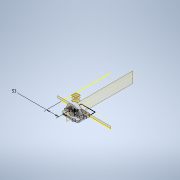
# Autodesk Inventor part: CameraHolder
Saved by Autodesk Inventor 2022 (Build 260153000, 153)
## iProperties
Created: 2024-03-25
Part Number: CameraHolder
Material: Generic
Document SubType Name: Modeling
Designer: Gotham City
Density: 1 g/cm^3
Appearance: Default
Author: Gotham City
Autodesk Inventor part; units mm, degrees
ref_plane "XY Plane" through (0, 0, 0) normal (0, 0, 1) x (1, 0, 0)
ref_plane "GlassTop" through (0, 0, 0) normal (0, 1, 0) x (-1, 0, 0)
ref_plane "CameraFocus" through (0, 1.5, 0) normal (0, 1, 0) x (-1, 0, 0)
ref_plane "HeatbedMountTop" through (0, -18, 0) normal (0, 1, 0) x (-1, 0, 0)
ref_plane "HeatbedBottom" through (0, -8, 0) normal (0, 1, 0) x (-1, 0, 0)
ref_plane "CameraBottom" through (0, -18.5, 0) normal (0, 1, 0) x (-1, 0, 0)
sketch "Sketch1" plane through (0, -18, 0) normal (0, 1, 0) x (-1, 0, 0)
  line L0 (-144, 0) -> (0, 0)
  line L1 (0, 0) -> (0, -144)
  line L2 (0, -144) -> (-144, -144)
  line L3 (-144, -144) -> (-144, 0)
  circle A0 centre (-11, -11) radius 2.5
  line L4 (-39.5, -4) -> (-24, -4)
  line L5 (-24, -4) -> (-24, -11.5)
  line L6 (-24, -11.5) -> (-39.5, -11.5)
  line L7 (-39.5, -11.5) -> (-39.5, -4)
  line L8 (-59.5, -4) -> (-44, -4)
  line L9 (-44, -4) -> (-44, -11.5)
  line L10 (-44, -11.5) -> (-59.5, -11.5)
  line L11 (-59.5, -11.5) -> (-59.5, -4)
  line L12 (-79.5, -4) -> (-64, -4)
  line L13 (-64, -4) -> (-64, -11.5)
  line L14 (-64, -11.5) -> (-79.5, -11.5)
  line L15 (-79.5, -11.5) -> (-79.5, -4)
  line L16 (-15.5, -44) -> (-8, -44)
  line L17 (-8, -44) -> (-8, -59.5)
  line L18 (-8, -59.5) -> (-15.5, -59.5)
  line L19 (-15.5, -59.5) -> (-15.5, -44)
  line L20 (-15.5, -79.5) -> (-15.5, -64)
  line L21 (-8, -64) -> (-8, -79.5)
  line L22 (-8, -79.5) -> (-15.5, -79.5)
  line L23 (-15.5, -64) -> (-8, -64)
  line L24 (-15.5, -99.5) -> (-15.5, -84)
  line L25 (-8, -84) -> (-8, -99.5)
  line L26 (-8, -99.5) -> (-15.5, -99.5)
  line L27 (-15.5, -84) -> (-8, -84)
  circle A1 centre (-11, -35) radius 2.5
  point P0 (0, 0)
  dimension "d5" = 144
  dimension "d6" = 144
  dimension "d7" = 11
  dimension "d8" = 11
  dimension "d9" = 5
  dimension "d10" = 7.5
  dimension "d11" = 15.5
  dimension "d12" = 4
  dimension "d13" = 24
  dimension "d16" = 20
  dimension "d21" = 7.5
  dimension "d22" = 15.5
  dimension "d23" = 8
  dimension "d24" = 44
  dimension "d27" = 20
  dimension "d32" = 5
  dimension "d33" = 24
  constraints: 56 end point, 6 parallel, 4 horizontal, 3 perpendicular, 2 centre point, 2 collinear, 1 coincident, 1 vertical, 1 vertical alignment, 30 other
  measures "d5" distance of L0.start L0.end
  measures "d6" distance of L0.end L1.end
  measures "d7" distance from line of L0 A0.centre
  measures "d8" distance from line of L1 A0.centre
  measures "d9" diameter of A0
  measures "d10" distance of L6.end L4.start
  measures "d11" distance of L4.start L4.end
  measures "d12" distance between parallel lines of L0 L4
  measures "d13" distance between parallel lines of L1 L5
  measures "d16" distance of L4.start L8.start
  measures "d21" distance of L16.start L16.end
  measures "d22" distance of L16.end L17.end
  measures "d23" distance between parallel lines of L1 L17
  measures "d24" distance between parallel lines of L0 L16
  measures "d27" distance of L16.start L20.end
  measures "d32" diameter of A1
  measures "d33" distance of A0.centre A1.centre
extrude "Extrusion1" add sketch "Sketch1" against normal blind 2
sketch "Sketch2" plane through (0, 0, 0) normal (0, 1, 0) x (-1, 0, 0)
  line L0 (30.5, -184.5) -> (-184.5, -184.5)
  line L1 (-184.5, -184.5) -> (-184.5, 30.5)
  line L2 (-184.5, 30.5) -> (30.5, 30.5)
  line L3 (30.5, 30.5) -> (30.5, -184.5)
  circle A0 centre (-11, -11) radius 2.5 construction
  point P0 (0, 0)
  dimension "d36" = 215
  dimension "d37" = 215
  dimension "d38" = 41.5
  dimension "d39" = 41.5
  constraints: 8 end point, 2 parallel, 1 horizontal, 1 perpendicular
  measures "d36" distance of L0.end L1.end
  measures "d37" distance of L0.start L0.end
  measures "d38" distance from line of L2 A0.centre
  measures "d39" distance from line of L3 A0.centre
extrude "Extrusion2" add sketch "Sketch2" against normal up to surface (8 mm away) separate body
ref_plane "MaxCameraFront" through (-30.5, 0, 40.5) normal (0, 0, 1) x (1, 0, 0)
sketch "Sketch4" plane through (0, -20, 0) normal (0, 1, 0) x (-1, 0, 0)
  line L0 (-84.5, 0) -> (-22.5, 0) construction
  line L1 (-22.5, 0) -> (-22.5, 53.5)
  line L2 (-22.5, 53.5) -> (-84.5, 53.5)
  line L3 (-84.5, 53.5) -> (-84.5, 0)
  line L4 (-84.5, 0) -> (-84.5, 0) construction
  line L5 (-22.5, 0) -> (-84.5, 0)
  line L6 (-184.5, 30.5) -> (30.5, 30.5) projected
  line L7 (30.5, 30.5) -> (30.5, -184.5) projected
  circle A0 centre (-38, 44.5) radius 1.5
  circle A1 centre (-38, 33) radius 1.5
  circle A2 centre (-76, 44.5) radius 1.5
  circle A3 centre (-76, 33) radius 1.5
  line L8 (-53.5, 53.5) -> (-53.5, 0) construction
  line L9 (-144, 0) -> (0, 0) construction
  dimension "d58" = 23
  dimension "d59" = 53
  dimension "d60" = 62
  dimension "d61" = 14
  dimension "d62" = 11.5
  dimension "d63" = 3
  dimension "d64" = 3
  dimension "d65" = 15.5
  dimension "d66" = 3
  dimension "d67" = 38
  dimension "d68" = 3
  constraints: 14 end point, 4 centre point, 3 perpendicular, 2 horizontal, 2 horizontal alignment, 2 point on line, 2 vertical alignment, 1 midpoint, 1 parallel, 1 vertical
  measures "d58" distance between parallel lines of L6 L2
  measures "d59" distance between parallel lines of L7 L1
  measures "d60" distance between parallel lines of L3 L1
  measures "d61" distance from line of L6 A0.centre
  measures "d62" distance of A0.centre A1.centre
  measures "d63" diameter of A0
  measures "d64" diameter of A1
  measures "d65" distance from line of L1 A0.centre
  measures "d66" diameter of A2
  measures "d67" distance of A0.centre A2.centre
  measures "d68" diameter of A3
extrude "Extrusion3" add sketch "Sketch4" against normal blind 3 separate body
ref_plane "CameraSideCenter" through (53.5, -20, 53.5) normal (1, 0, 0) x (0, 1, 0)
sketch "Sketch3" plane through (53.5, 0, -184.5) normal (-1, 0, 0) x (0, 0, 1)
  line L0 (-53, 1.5) -> (318, 1.5) construction
  line L1 (225, 29.8) -> (225, -28.3) construction
  circle A0 centre (245, 1.5) radius 20 construction
  line L2 (245, 21.5) -> (245, -18.5)
  arc A1 (245, 21.5) -> (245, -18.5) centre (245, 1.5) ccw
  point P0 (184.5, 0)
  dimension "d47" = 40
  constraints: 4 point on circle, 2 centre point, 2 end point, 2 tangent, 1 midpoint, 1 point on line, 1 vertical
  measures "d47" diameter of A0
revolve "Revolution1" add sketch "Sketch3" angle 360 about axis through (53.5, 21.5, 60.5) along (0, -1, 0) separate body
sketch "Sketch6" plane through (0, -20, 0) normal (0, 1, 0) x (1, 0, 0)
  line L0 (17.5, -81.5) -> (89.5, -81.5)
  line L1 (89.5, -81.5) -> (89.5, -25.5)
  line L2 (89.5, -25.5) -> (17.5, -25.5)
  line L3 (17.5, -25.5) -> (17.5, -81.5)
  circle A0 centre (53.5, -60.5) radius 20 construction
  circle A1 centre (38, -33) radius 1.5 construction
  line L4 (33.5, -81.5) -> (33.5, -25.5) construction
  line L5 (73.5, -81.5) -> (73.5, -25.5) construction
  line L6 (17.5, -31.5) -> (89.5, -31.5) construction
  line L7 (17.5, -80.5) -> (95.4239, -80.5) construction
  point P0 (0, 0)
  dimension "d69" = 16
  dimension "d70" = 16
  dimension "d71" = 1
  dimension "d72" = 6
  constraints: 16 end point, 7 point on line, 5 perpendicular, 4 tangent, 2 parallel, 1 horizontal
  measures "d69" distance between parallel lines of L3 L4
  measures "d70" distance between parallel lines of L1 L5
  measures "d71" distance between parallel lines of L7 L0
  measures "d72" distance between parallel lines of L6 L2
extrude "Extrusion5" add sketch "Sketch6" along normal blind 8 separate body
revolve "Revolution3" cut sketch "Sketch3" angle 360 about axis through (53.5, 21.5, 60.5) along (0, -1, 0) bodies 5
sketch "Sketch7" plane through (0, -12, 0) normal (0, 1, 0) x (1, 0, 0)
  circle A0 centre (76, -44.5) radius 1.5 projected
  circle A1 centre (76, -33) radius 1.5 projected
  circle A2 centre (38, -44.5) radius 1.5 projected
  circle A3 centre (38, -33) radius 1.5 projected
  point P0 (0, 0)
hole "Hole1" at (76, -12, 33) at (76, -12, 44.5) at (38, -12, 44.5) at (38, -12, 33) direction (0, -1, 0) diameter 2.6 end through all counterbore diameter 5.5 counterbore depth 2 bodies 5 clearance for "Socket Head Cap Screw ISO 4762" size "M2.5" standard "ISO"
sketch "Sketch8" plane through (0, -12, 0) normal (0, 1, 0) x (1, 0, 0)
  line L0 (17.5, -25.5) -> (17.5, -81.5) construction
  line L1 (89.5, -81.5) -> (89.5, -25.5) construction
  line L2 (89.5, -81.5) -> (89.5, -25.5) projected
  line L3 (17.5, -52.5) -> (89.5, -52.5)
  line L4 (89.5, -52.5) -> (89.5, -68.5)
  line L5 (89.5, -68.5) -> (17.5, -68.5)
  line L6 (17.5, -68.5) -> (17.5, -52.5)
  circle A0 centre (53.5, -60.5) radius 20 construction
  line L7 (53.5, -60.5) -> (89.5, -60.5) construction
  point P0 (0, 0)
  dimension "d83" = 16
  constraints: 10 end point, 2 horizontal, 2 parallel, 2 point on line, 1 midpoint, 1 perpendicular
  measures "d83" distance between parallel lines of L5 L3
extrude "Extrusion6" add sketch "Sketch8" along normal blind 40 separate body
revolve "Revolution4" cut sketch "Sketch3" angle 360 about axis through (53.5, 21.5, 60.5) along (0, -1, 0) bodies 6
sketch "Sketch9" plane through (17.5, 28, 68.5) normal (0, 0, 1) x (1, 0, 0)
  arc A0 (48.3996, -40) -> (23.6004, -40) centre (36, -26.5) ccw construction
  line L0 (55.75, -40) -> (61.25, -40) projected
  line L1 (36, -26.5) -> (54.3303, -26.5)
  line L2 (54.3303, -26.5) -> (54.3303, -40)
  line L3 (54.3303, -40) -> (36, -40)
  line L4 (36, -40) -> (36, -26.5) construction
  line L5 (36, -26.5) -> (17.6697, -26.5)
  line L6 (17.6697, -26.5) -> (17.6697, -40)
  line L7 (17.6697, -40) -> (36, -40)
  point P0 (-17.5, -28)
  point P1 (55.75, -40)
  constraints: 14 end point, 2 parallel, 2 symmetric about line, 1 horizontal, 1 perpendicular, 1 point on circle, 1 point on line
extrude "Extrusion7" cut sketch "Sketch9" against normal through all bodies 6
sketch "Sketch10" plane through (17.5, 28, 68.5) normal (0, 0, 1) x (1, 0, 0)
  arc A0 (48.3996, -40) -> (23.6004, -40) centre (36, -26.5) ccw construction
  arc A1 (62.3303, -26.5) -> (9.6697, -26.5) centre (36, -26.5) ccw
  line L0 (0, -40) -> (0, 0) projected
  line L1 (0, -32) -> (0, 0)
  line L2 (0, 0) -> (72, 0) projected
  line L3 (36, 1.8) -> (36, -56.3) construction
  line L4 (72, -32) -> (72, 0)
  line L5 (9.6697, -26.5) -> (9.6697, -32)
  line L6 (9.6697, -32) -> (0, -32)
  line L7 (62.3303, -26.5) -> (62.3303, -32)
  line L8 (62.3303, -32) -> (72, -32)
  line L9 (0, -40) -> (72, -40) projected
  point P0 (-17.5, -28)
  point P1 (17.6697, -26.5)
  point P2 (54.3303, -26.5)
  dimension "d89" = 8
  dimension "d90" = 8
  constraints: 12 end point, 3 symmetric about line, 2 point on circle, 1 centre point, 1 coincident, 1 collinear, 1 perpendicular, 1 point on line, 1 tangent, 1 vertical
  measures "d89" distance of L5.start point (17.67, -26.5)
  measures "d90" distance between parallel lines of L9 L6
extrude "Extrusion8" cut sketch "Sketch10" against normal through all bodies 6
sketch "Sketch11" plane through (17.5, -4, 68.5) normal (0, 1, 0) x (1, 0, 0)
  line L0 (0, 16) -> (9.6697, 16) construction
  line L1 (9.6697, 0) -> (0, 0) construction
  line L2 (72, 16) -> (0, 16) construction
  line L3 (0, 16) -> (9.6697, 0) construction
  line L4 (0, 0) -> (17.6697, 0) construction
  line L5 (0, 0) -> (9.6697, 16) construction
  circle A0 centre (4.8348, 8) radius 1.5
  line L6 (36, 306) -> (36, -65) construction
  circle A1 centre (67.1652, 8) radius 1.5
  point P0 (-17.5, 68.5)
  point P1 (17.6697, 16)
  point P2 (27.6004, 0)
  dimension "d94" = 3
  constraints: 4 end point, 2 centre point, 1 coincident, 1 midpoint, 1 symmetric about line, 1 other
  measures "d94" diameter of A0
hole "Hole2" at (22.3348, -4, 60.5) at (84.6652, -4, 60.5) direction (0, -1, 0) diameter 2.6 end through all counterbore diameter 5.5 counterbore depth 2 bodies 6 5 clearance for "Socket Head Cap Screw ISO 4762" size "M2.5" standard "ISO"
fillet "Fillet1" radius 8 2 edges at (17.5, -16, 81.5) (89.5, -16, 81.5)
ref_plane "Work Plane9" through (22.3348, -16, 60.5) normal (0, 1, 0) x (1, 0, 0)
sketch "Sketch12" plane through (22.3348, -16, 60.5) normal (0, 1, 0) x (1, 0, 0)
  circle A0 centre (0, 0) radius 1.3 construction
  circle A1 centre (0, 0) radius 1.3 construction
  line L0 (1.4722, 2.55) -> (2.9445, 0)
  line L1 (2.9445, 0) -> (1.4722, -2.55)
  line L2 (1.4722, -2.55) -> (-1.4722, -2.55)
  line L3 (-1.4722, -2.55) -> (-2.9445, 0) construction
  line L4 (-2.9445, 0) -> (-1.4722, 2.55) construction
  line L5 (-1.4722, 2.55) -> (1.4722, 2.55)
  line L6 (-1.4722, 2.55) -> (-4.8348, 2.55)
  line L7 (-4.8348, 8) -> (-4.8348, -8) construction
  line L8 (-1.4722, -2.55) -> (-4.8348, -2.55)
  line L9 (-4.8348, 2.55) -> (-4.8348, -2.55)
  line L10 (31.1652, 298) -> (31.1652, -73) construction
  point P0 (-22.3348, 60.5)
  dimension "d105" = 5.1
  constraints: 18 end point, 2 horizontal, 2 point on line, 1 coincident, 1 collinear, 1 perpendicular, 13 other
  measures "d105" distance between parallel lines of L2 L5
extrude "Extrusion9" cut sketch "Sketch12" along normal blind 2.1 bodies 5
mirror "Mirror1" about plane through (53.5, -20, 53.5) normal (1, 0, 0) of "Extrusion9" bodies 5
thicken "Thicken1" operation add thickness 0.5 both sides no extend neighbours yes toward (0, 1, 0) bodies 6 faces at (31.3216, -12, 60.4478)
thicken "Thicken2" operation add thickness 0.5 both sides no extend neighbours yes toward (0, 1, 0) bodies 6 faces at (75.6784, -12, 60.4478)
fillet "Fillet3" radius 2 6 edges at (17.5, -4, 60.5) (89.5, -4, 60.5) (27.1697, -4, 60.5) (79.8303, -4, 60.5) (35.1697, -11.5, 60.5) (71.8303, -11.5, 60.5)
fillet "Fillet4" radius 4 2 edges at (89.5, -16, 25.5) (17.5, -16, 25.5)
equation "\"d21\" = d10"
equation "\"d22\" = d11"
equation "\"d64\" = d63"
equation "\"d66\" = d63"
equation "\"d68\" = d63"
equation "\"d69\" = d70"
equation "\"d90\" = d89"
body "Solid1"
body "Solid2"
body "Solid3"
body "Solid4"
body "Solid5"
body "Solid6"
